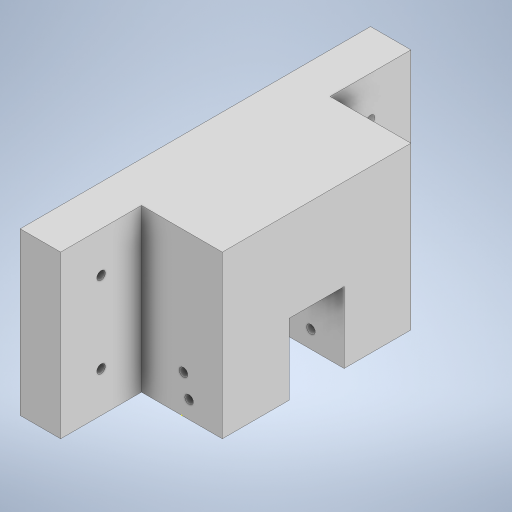
# Autodesk Inventor part: ハンド_簡易4
Saved by Autodesk Inventor 2023 (Build 270158000, 158)
## iProperties
Created: 2022-04-27
Part Number: ハンド_簡易4
Material: 一般
Document SubType Name: Modeling
Designer: yuta
Density: 1 g/cm^3
Appearance: 既定
Author: yuta
Autodesk Inventor part; units mm, degrees
ref_plane "YZ Plane" through (0, 0, 0) normal (1, 0, 0) x (0, 1, 0)
ref_plane "XZ Plane" through (0, 0, 0) normal (0, 1, 0) x (-1, 0, 0)
ref_plane "XY Plane" through (0, 0, 0) normal (0, 0, 1) x (1, 0, 0)
sketch "スケッチ1" plane through (0, 0, 0) normal (0, 1, 0) x (-1, 0, 0)
  line L0 (0, 0) -> (30, 0)
  line L1 (30, 0) -> (30, -130)
  line L2 (30, -130) -> (0, -130)
  line L3 (0, -130) -> (0, 0)
  dimension "d0" = 30
  dimension "d1" = 130
  constraints: 8 end point, 2 parallel, 1 horizontal, 1 perpendicular
  measures "d0" distance of L1.end L2.end
  measures "d1" distance of L0.end L1.end
extrude "押し出し1" add sketch "スケッチ1" along normal blind 60
sketch "スケッチ2" plane through (0, 60, 0) normal (0, 1, 0) x (1, 0, 0)
  line L0 (-30, 0) -> (0, 0) projected
  line L1 (0, 0) -> (-15, 0)
  line L2 (-15, 0) -> (-15, 30)
  line L3 (-15, 30) -> (0, 30)
  line L4 (0, 30) -> (0, 0)
  line L5 (0, 130) -> (-30, 130) projected
  line L6 (0, 130) -> (-15, 130)
  line L7 (-15, 130) -> (-15, 100)
  line L8 (-15, 100) -> (0, 100)
  line L9 (0, 100) -> (0, 130)
  dimension "d4" = 15
  dimension "d5" = 30
  dimension "d6" = 15
  dimension "d7" = 30
  constraints: 16 end point, 4 parallel, 2 horizontal, 2 perpendicular
  measures "d4" distance of L2.end L3.end
  measures "d5" distance of L1.end L2.end
  measures "d6" distance of L8.end L7.end
  measures "d7" distance of L7.end L6.end
extrude "押し出し2" cut sketch "スケッチ2" against normal blind 60
sketch "スケッチ4" plane through (0, 0, -30) normal (1, 0, 0) x (0, 0, -1)
  line L0 (0, 0) -> (70, 0) projected
  line L1 (70, 60) -> (70, 0) projected
  line L2 (0, 0) -> (70, 0)
  line L3 (70, 0) -> (70, 60)
  line L4 (70, 60) -> (0, 60)
  line L5 (0, 60) -> (0, 0)
  point P0 (-30, 0)
  constraints: 8 end point, 2 parallel, 1 horizontal, 1 perpendicular
extrude "押し出し3" add sketch "スケッチ4" along normal blind 15
sketch "スケッチ5" plane through (-15, 0, -30) normal (0, 0, 1) x (1, 0, 0)
  line L0 (30, 0) -> (0, 0) projected
  line L1 (9.0427, 0) -> (3.8663, 19.3185)
  line L2 (9.0427, 0) -> (29.0427, 0) construction
  line L3 (3.8663, 19.3185) -> (30, 26.321)
  line L4 (30, 26.321) -> (30, 0)
  line L5 (30, 0) -> (9.0427, 0)
  point P0 (15, 0)
  dimension "d15" = 20
  dimension "d16" = 105
  constraints: 10 end point, 2 perpendicular, 1 collinear, 1 equal length, 1 horizontal, 1 point on line
  measures "d15" distance of L1.start L1.end
  measures "d16" angle of L2 L1
extrude "押し出し4" cut sketch "スケッチ5" against normal blind 45.2
sketch "スケッチ6" plane through (-15, 0, -30) normal (0, 0, 1) x (1, 0, 0)
  line L0 (9.0427, 0) -> (3.8663, 19.3185) projected
  line L1 (3.8663, 19.3185) -> (9.0427, 0)
  line L2 (0, 0) -> (30, 0) projected
  line L3 (9.0427, 0) -> (30, 0)
  line L4 (30, 26.321) -> (30, 0) projected
  line L5 (30, 0) -> (30, 26.321)
  line L6 (30, 26.321) -> (3.8663, 19.3185)
  point P0 (15, 0)
  constraints: 8 end point, 2 collinear, 2 perpendicular
extrude "押し出し5" add sketch "スケッチ6" against normal blind 24.8
sketch "スケッチ7" plane through (-15, 0, -30) normal (0, 0, 1) x (1, 0, 0)
  point P0 (15, 0)
sketch "スケッチ8" plane through (-15, 0, -75.2) normal (0, 0, 1) x (1, 0, 0)
  line L0 (9.0427, 0) -> (3.8663, 19.3185) projected
  line L1 (3.8663, 19.3185) -> (30, 26.321) projected
  circle A0 centre (15.5961, 14.1793) radius 1.6
  circle A1 centre (17.6666, 6.4519) radius 1.6
  point P0 (15, 0)
  dimension "d21" = 10
  dimension "d22" = 8
  dimension "d23" = 10
  dimension "d24" = 16
  dimension "d25" = 3.2
  dimension "d26" = 3.2
  constraints: 2 centre point, 2 coincident
  measures "d21" distance from line of point (15.596, 14.179) L0
  measures "d22" distance from line of point (15.596, 14.179) L1
  measures "d23" distance from line of point (17.667, 6.452) L0
  measures "d24" distance from line of point (17.667, 6.452) L1
  measures "d25" diameter of A0
  measures "d26" diameter of A1
extrude "押し出し6" cut sketch "スケッチ8" along normal mid plane 100
sketch "スケッチ9" plane through (-15, 60, 0) normal (1, 0, 0) x (0, 0, -1)
  line L0 (0, 0) -> (30, 0) projected
  line L1 (0, -60) -> (0, 0) projected
  line L2 (100, 0) -> (130, 0) projected
  line L3 (130, 0) -> (130, -60) projected
  point P0 (15, -15)
  point P1 (15, -45)
  point P2 (115, -15)
  point P3 (115, -45)
  dimension "d29" = 15
  dimension "d30" = 15
  dimension "d31" = 15
  dimension "d32" = 45
  dimension "d33" = 15
  dimension "d34" = 15
  dimension "d35" = 30
  dimension "d36" = 15
  measures "d29" distance from line of point (15, -15) L0
  measures "d30" distance from line of L1 point (15, -15)
  measures "d31" distance from line of L1 point (15, -45)
  measures "d32" distance from line of L0 point (15, -45)
  measures "d33" distance from line of L2 point (115, -15)
  measures "d34" distance from line of L3 point (115, -15)
  measures "d35" distance of point (115, -15) point (115, -45)
  measures "d36" distance from line of L3 point (115, -45)
hole "穴1" at (-15, 45, -15) at (-15, 15, -15) at (-15, 45, -115) at (-15, 15, -115) direction (-1, 0, 0) diameter 3.2 end through all
